Autodesk Fusion 360 part; units mm, degrees
note: some values were not read from the file. Chosen so that the rebuilt part matches the saved one: a direction. Set by a fixed rule: which sketch regions a step uses; which face or edge a step refers to.
(part 4 of 6)
  line L915 (71.0316, -22.4896) -> (71.0316, -29.1571)
  line L916 (71.6269, -30.7446) -> (71.6269, -26.6171)
  line L917 (71.6269, -25.0296) -> (71.6269, -18.3621)
  line L918 (71.6269, -16.7746) -> (71.6269, -10.1071)
  line L919 (71.6269, -8.5196) -> (71.6269, -4.3921)
  line L920 (72.2223, -5.9796) -> (72.2223, -12.6471)
  line L921 (72.2223, -14.2346) -> (72.2223, -20.9021)
  line L922 (72.2223, -22.4896) -> (72.2223, -29.1571)
  line L923 (72.8176, -30.7446) -> (72.8176, -26.6171)
  line L924 (72.8176, -25.0296) -> (72.8176, -18.3621)
  line L925 (72.8176, -16.7746) -> (72.8176, -10.1071)
  line L926 (72.8176, -8.5196) -> (72.8176, -4.3921)
  line L927 (73.4129, -5.9796) -> (73.4129, -12.6471)
  line L928 (73.4129, -14.2346) -> (73.4129, -20.9021)
  line L929 (73.4129, -22.4896) -> (73.4129, -29.1571)
  line L930 (74.0082, -30.7446) -> (74.0082, -26.6171)
  line L931 (74.0082, -25.0296) -> (74.0082, -18.3621)
  line L932 (74.0082, -16.7746) -> (74.0082, -10.1071)
  line L933 (74.0082, -8.5196) -> (74.0082, -4.3921)
  line L934 (74.6035, -5.9796) -> (74.6035, -12.6471)
  line L935 (74.6035, -14.2346) -> (74.6035, -20.9021)
  line L936 (74.6035, -22.4896) -> (74.6035, -29.1571)
  line L937 (75.1988, -30.7446) -> (75.1988, -26.6171)
  line L938 (75.1988, -25.0296) -> (75.1988, -18.3621)
  line L939 (75.1988, -16.7746) -> (75.1988, -10.1071)
  line L940 (75.1988, -8.5196) -> (75.1988, -4.3921)
  line L941 (75.7941, -5.9796) -> (75.7941, -12.6471)
  line L942 (75.7941, -14.2346) -> (75.7941, -20.9021)
  line L943 (75.7941, -22.4896) -> (75.7941, -29.1571)
  line L944 (76.3894, -30.7446) -> (76.3894, -26.6171)
  line L945 (76.3894, -25.0296) -> (76.3894, -18.3621)
  line L946 (76.3894, -16.7746) -> (76.3894, -10.1071)
  line L947 (76.3894, -8.5196) -> (76.3894, -4.3921)
  line L948 (76.9848, -5.9796) -> (76.9848, -12.6471)
  line L949 (76.9848, -14.2346) -> (76.9848, -20.9021)
  line L950 (76.9848, -22.4896) -> (76.9848, -29.1571)
  line L951 (77.5801, -30.7446) -> (77.5801, -26.6171)
  line L952 (77.5801, -25.0296) -> (77.5801, -18.3621)
  line L953 (77.5801, -16.7746) -> (77.5801, -10.1071)
  line L954 (77.5801, -8.5196) -> (77.5801, -4.3921)
  line L955 (78.1754, -5.9796) -> (78.1754, -12.6471)
  line L956 (78.1754, -14.2346) -> (78.1754, -20.9021)
  line L957 (78.1754, -22.4896) -> (78.1754, -29.1571)
  line L958 (78.7707, -30.7446) -> (78.7707, -26.6171)
  line L959 (78.7707, -25.0296) -> (78.7707, -18.3621)
  line L960 (78.7707, -16.7746) -> (78.7707, -10.1071)
  line L961 (78.7707, -8.5196) -> (78.7707, -4.3921)
  line L962 (79.366, -5.9796) -> (79.366, -12.6471)
  line L963 (79.366, -14.2346) -> (79.366, -20.9021)
  line L964 (79.366, -22.4896) -> (79.366, -29.1571)
  line L965 (79.9613, -30.7446) -> (79.9613, -26.6171)
  line L966 (79.9613, -25.0296) -> (79.9613, -18.3621)
  line L967 (79.9613, -16.7746) -> (79.9613, -10.1071)
  line L968 (79.9613, -8.5196) -> (79.9613, -4.3921)
  line L969 (80.5566, -5.9796) -> (80.5566, -12.6471)
  line L970 (80.5566, -14.2346) -> (80.5566, -20.9021)
  line L971 (80.5566, -22.4896) -> (80.5566, -29.1571)
  line L972 (81.1519, -30.7446) -> (81.1519, -26.6171)
  line L973 (81.1519, -25.0296) -> (81.1519, -18.3621)
  line L974 (81.1519, -16.7746) -> (81.1519, -10.1071)
  line L975 (81.1519, -8.5196) -> (81.1519, -4.3921)
  line L976 (81.7473, -5.9796) -> (81.7473, -12.6471)
  line L977 (81.7473, -14.2346) -> (81.7473, -20.9021)
  line L978 (81.7473, -22.4896) -> (81.7473, -29.1571)
  line L979 (82.3426, -30.7446) -> (82.3426, -26.6171)
  line L980 (82.3426, -25.0296) -> (82.3426, -18.3621)
  line L981 (82.3426, -16.7746) -> (82.3426, -10.1071)
  line L982 (82.3426, -8.5196) -> (82.3426, -4.3921)
  line L983 (82.9379, -5.9796) -> (82.9379, -12.6471)
  line L984 (82.9379, -14.2346) -> (82.9379, -20.9021)
  line L985 (82.9379, -22.4896) -> (82.9379, -29.1571)
  line L986 (83.5332, -30.7446) -> (83.5332, -26.6171)
  line L987 (83.5332, -25.0296) -> (83.5332, -18.3621)
  line L988 (83.5332, -16.7746) -> (83.5332, -10.1071)
  line L989 (83.5332, -8.5196) -> (83.5332, -4.3921)
  line L990 (84.1285, -5.9796) -> (84.1285, -12.6471)
  line L991 (84.1285, -14.2346) -> (84.1285, -20.9021)
  line L992 (84.1285, -22.4896) -> (84.1285, -29.1571)
  line L993 (84.7238, -30.7446) -> (84.7238, -26.6171)
  line L994 (84.7238, -25.0296) -> (84.7238, -18.3621)
  line L995 (84.7238, -16.7746) -> (84.7238, -10.1071)
  line L996 (84.7238, -8.5196) -> (84.7238, -4.3921)
  line L997 (85.3191, -5.9796) -> (85.3191, -12.6471)
  line L998 (85.3191, -14.2346) -> (85.3191, -20.9021)
  line L999 (85.3191, -22.4896) -> (85.3191, -29.1571)
  line L1000 (85.9144, -30.7446) -> (85.9144, -26.6171)
  line L1001 (85.9144, -25.0296) -> (85.9144, -18.3621)
  line L1002 (85.9144, -16.7746) -> (85.9144, -10.1071)
  line L1003 (85.9144, -8.5196) -> (85.9144, -4.3921)
  line L1004 (86.5098, -5.9796) -> (86.5098, -12.6471)
  line L1005 (86.5098, -14.2346) -> (86.5098, -20.9021)
  line L1006 (86.5098, -22.4896) -> (86.5098, -29.1571)
  line L1007 (87.1051, -30.7446) -> (87.1051, -26.6171)
  line L1008 (87.1051, -25.0296) -> (87.1051, -18.3621)
  line L1009 (87.1051, -16.7746) -> (87.1051, -10.1071)
  line L1010 (87.1051, -8.5196) -> (87.1051, -4.3921)
  line L1011 (87.7004, -5.9796) -> (87.7004, -12.6471)
  line L1012 (87.7004, -14.2346) -> (87.7004, -20.9021)
  line L1013 (87.7004, -22.4896) -> (87.7004, -29.1571)
  line L1014 (88.2957, -30.7446) -> (88.2957, -26.6171)
  line L1015 (88.2957, -25.0296) -> (88.2957, -18.3621)
  line L1016 (88.2957, -16.7746) -> (88.2957, -10.1071)
  line L1017 (88.2957, -8.5196) -> (88.2957, -4.3921)
  line L1018 (88.891, -5.9796) -> (88.891, -12.6471)
  line L1019 (88.891, -14.2346) -> (88.891, -20.9021)
  line L1020 (88.891, -22.4896) -> (88.891, -29.1571)
  line L1021 (89.4863, -30.7446) -> (89.4863, -26.6171)
  line L1022 (89.4863, -25.0296) -> (89.4863, -18.3621)
  line L1023 (89.4863, -16.7746) -> (89.4863, -10.1071)
  line L1024 (89.4863, -8.5196) -> (89.4863, -4.3921)
  line L1025 (90.0816, -5.9796) -> (90.0816, -12.6471)
  line L1026 (90.0816, -14.2346) -> (90.0816, -20.9021)
  line L1027 (90.0816, -22.4896) -> (90.0816, -29.1571)
  line L1028 (90.6769, -30.7446) -> (90.6769, -26.6171)
  line L1029 (90.6769, -25.0296) -> (90.6769, -18.3621)
  line L1030 (90.6769, -16.7746) -> (90.6769, -10.1071)
  line L1031 (90.6769, -8.5196) -> (90.6769, -4.3921)
  line L1032 (91.2723, -5.9796) -> (91.2723, -12.6471)
  line L1033 (91.2723, -14.2346) -> (91.2723, -20.9021)
  line L1034 (91.2723, -22.4896) -> (91.2723, -29.1571)
  line L1035 (91.8676, -30.7446) -> (91.8676, -26.6171)
  line L1036 (91.8676, -25.0296) -> (91.8676, -18.3621)
  line L1037 (91.8676, -16.7746) -> (91.8676, -10.1071)
  line L1038 (91.8676, -8.5196) -> (91.8676, -4.3921)
  line L1039 (93.7503, -30.7446) -> (95.3378, -30.7446)
  spline S766 degree 3 poles (95.3378, -30.7446) (95.3524, -30.7446) (95.3643, -30.7327) (95.3643, -30.7181) knots 0 0 0 0 1 1 1 1
  line L1040 (95.3643, -30.7181) -> (95.3643, -6.006)
  spline S767 degree 3 poles (95.3643, -6.006) (95.3643, -5.9915) (95.3524, -5.9796) (95.3378, -5.9796) knots 0 0 0 0 1 1 1 1
  line L1041 (95.3378, -5.9796) -> (93.7503, -5.9796)
  spline S768 degree 3 poles (93.7503, -5.9796) (93.7358, -5.9796) (93.7239, -5.9915) (93.7239, -6.006) knots 0 0 0 0 1 1 1 1
  line L1042 (93.7239, -6.006) -> (93.7239, -6.4294)
  spline S769 degree 3 poles (93.7239, -6.4294) (93.7239, -6.4558) (93.7503, -6.4294) (93.7239, -6.4294) knots 0 0 0 0 1 1 1 1
  line L1043 (93.7239, -6.4294) -> (92.9566, -6.4294)
  spline S770 degree 3 poles (92.9566, -6.4294) (92.942, -6.4294) (92.9301, -6.4413) (92.9301, -6.4558) knots 0 0 0 0 1 1 1 1
  line L1044 (92.9301, -6.4558) -> (92.9301, -8.0433)
  spline S771 degree 3 poles (92.9301, -8.0433) (92.9301, -8.0579) (92.942, -8.0698) (92.9566, -8.0698) knots 0 0 0 0 1 1 1 1
  line L1045 (92.9566, -8.0698) -> (93.7239, -8.0698)
  spline S772 degree 3 poles (93.7239, -8.0698) (93.7503, -8.0698) (93.7239, -8.0433) (93.7239, -8.0698) knots 0 0 0 0 1 1 1 1
  line L1046 (93.7239, -8.0698) -> (93.7239, -9.6044)
  spline S773 degree 3 poles (93.7239, -9.6044) (93.7239, -9.6308) (93.7503, -9.6044) (93.7239, -9.6044) knots 0 0 0 0 1 1 1 1
  line L1047 (93.7239, -9.6044) -> (92.9566, -9.6044)
  spline S774 degree 3 poles (92.9566, -9.6044) (92.942, -9.6044) (92.9301, -9.6163) (92.9301, -9.6308) knots 0 0 0 0 1 1 1 1
  line L1048 (92.9301, -9.6308) -> (92.9301, -11.2183)
  spline S775 degree 3 poles (92.9301, -11.2183) (92.9301, -11.2329) (92.942, -11.2448) (92.9566, -11.2448) knots 0 0 0 0 1 1 1 1
  line L1049 (92.9566, -11.2448) -> (93.7239, -11.2448)
  spline S776 degree 3 poles (93.7239, -11.2448) (93.7503, -11.2448) (93.7239, -11.2183) (93.7239, -11.2448) knots 0 0 0 0 1 1 1 1
  line L1050 (93.7239, -11.2448) -> (93.7239, -12.7794)
  spline S777 degree 3 poles (93.7239, -12.7794) (93.7239, -12.8058) (93.7503, -12.7794) (93.7239, -12.7794) knots 0 0 0 0 1 1 1 1
  line L1051 (93.7239, -12.7794) -> (92.9566, -12.7794)
  spline S778 degree 3 poles (92.9566, -12.7794) (92.942, -12.7794) (92.9301, -12.7913) (92.9301, -12.8058) knots 0 0 0 0 1 1 1 1
  line L1052 (92.9301, -12.8058) -> (92.9301, -14.3933)
  spline S779 degree 3 poles (92.9301, -14.3933) (92.9301, -14.4079) (92.942, -14.4198) (92.9566, -14.4198) knots 0 0 0 0 1 1 1 1
  line L1053 (92.9566, -14.4198) -> (93.7239, -14.4198)
  spline S780 degree 3 poles (93.7239, -14.4198) (93.7503, -14.4198) (93.7239, -14.3933) (93.7239, -14.4198) knots 0 0 0 0 1 1 1 1
  line L1054 (93.7239, -14.4198) -> (93.7239, -15.9544)
  spline S781 degree 3 poles (93.7239, -15.9544) (93.7239, -15.9808) (93.7503, -15.9544) (93.7239, -15.9544) knots 0 0 0 0 1 1 1 1
  line L1055 (93.7239, -15.9544) -> (92.9566, -15.9544)
  spline S782 degree 3 poles (92.9566, -15.9544) (92.942, -15.9544) (92.9301, -15.9663) (92.9301, -15.9808) knots 0 0 0 0 1 1 1 1
  line L1056 (92.9301, -15.9808) -> (92.9301, -17.5683)
  spline S783 degree 3 poles (92.9301, -17.5683) (92.9301, -17.5829) (92.942, -17.5948) (92.9566, -17.5948) knots 0 0 0 0 1 1 1 1
  line L1057 (92.9566, -17.5948) -> (93.7239, -17.5948)
  spline S784 degree 3 poles (93.7239, -17.5948) (93.7503, -17.5948) (93.7239, -17.5683) (93.7239, -17.5948) knots 0 0 0 0 1 1 1 1
  line L1058 (93.7239, -17.5948) -> (93.7239, -19.1294)
  spline S785 degree 3 poles (93.7239, -19.1294) (93.7239, -19.1558) (93.7503, -19.1294) (93.7239, -19.1294) knots 0 0 0 0 1 1 1 1
  line L1059 (93.7239, -19.1294) -> (92.9566, -19.1294)
  spline S786 degree 3 poles (92.9566, -19.1294) (92.942, -19.1294) (92.9301, -19.1413) (92.9301, -19.1558) knots 0 0 0 0 1 1 1 1
  line L1060 (92.9301, -19.1558) -> (92.9301, -20.7433)
  spline S787 degree 3 poles (92.9301, -20.7433) (92.9301, -20.7579) (92.942, -20.7698) (92.9566, -20.7698) knots 0 0 0 0 1 1 1 1
  line L1061 (92.9566, -20.7698) -> (93.7239, -20.7698)
  spline S788 degree 3 poles (93.7239, -20.7698) (93.7503, -20.7698) (93.7239, -20.7433) (93.7239, -20.7698) knots 0 0 0 0 1 1 1 1
  line L1062 (93.7239, -20.7698) -> (93.7239, -22.3044)
  spline S789 degree 3 poles (93.7239, -22.3044) (93.7239, -22.3308) (93.7503, -22.3044) (93.7239, -22.3044) knots 0 0 0 0 1 1 1 1
  line L1063 (93.7239, -22.3044) -> (92.9566, -22.3044)
  spline S790 degree 3 poles (92.9566, -22.3044) (92.942, -22.3044) (92.9301, -22.3163) (92.9301, -22.3308) knots 0 0 0 0 1 1 1 1
  line L1064 (92.9301, -22.3308) -> (92.9301, -23.9183)
  spline S791 degree 3 poles (92.9301, -23.9183) (92.9301, -23.9329) (92.942, -23.9448) (92.9566, -23.9448) knots 0 0 0 0 1 1 1 1
  line L1065 (92.9566, -23.9448) -> (93.7239, -23.9448)
  spline S792 degree 3 poles (93.7239, -23.9448) (93.7503, -23.9448) (93.7239, -23.9183) (93.7239, -23.9448) knots 0 0 0 0 1 1 1 1
  line L1066 (93.7239, -23.9448) -> (93.7239, -25.4794)
  spline S793 degree 3 poles (93.7239, -25.4794) (93.7239, -25.5058) (93.7503, -25.4794) (93.7239, -25.4794) knots 0 0 0 0 1 1 1 1
  line L1067 (93.7239, -25.4794) -> (92.9566, -25.4794)
  spline S794 degree 3 poles (92.9566, -25.4794) (92.942, -25.4794) (92.9301, -25.4913) (92.9301, -25.5058) knots 0 0 0 0 1 1 1 1
  line L1068 (92.9301, -25.5058) -> (92.9301, -27.0933)
  spline S795 degree 3 poles (92.9301, -27.0933) (92.9301, -27.1079) (92.942, -27.1198) (92.9566, -27.1198) knots 0 0 0 0 1 1 1 1
  line L1069 (92.9566, -27.1198) -> (93.7239, -27.1198)
  spline S796 degree 3 poles (93.7239, -27.1198) (93.7503, -27.1198) (93.7239, -27.0933) (93.7239, -27.1198) knots 0 0 0 0 1 1 1 1
  line L1070 (93.7239, -27.1198) -> (93.7239, -28.6544)
  spline S797 degree 3 poles (93.7239, -28.6544) (93.7239, -28.6808) (93.7503, -28.6544) (93.7239, -28.6544) knots 0 0 0 0 1 1 1 1
  line L1071 (93.7239, -28.6544) -> (92.9566, -28.6544)
  spline S798 degree 3 poles (92.9566, -28.6544) (92.942, -28.6544) (92.9301, -28.6663) (92.9301, -28.6808) knots 0 0 0 0 1 1 1 1
  line L1072 (92.9301, -28.6808) -> (92.9301, -30.2683)
  spline S799 degree 3 poles (92.9301, -30.2683) (92.9301, -30.2829) (92.942, -30.2948) (92.9566, -30.2948) knots 0 0 0 0 1 1 1 1
  line L1073 (92.9566, -30.2948) -> (93.7239, -30.2948)
  spline S800 degree 3 poles (93.7239, -30.2948) (93.7503, -30.2948) (93.7239, -30.2683) (93.7239, -30.2948) knots 0 0 0 0 1 1 1 1
  line L1074 (93.7239, -30.2948) -> (93.7239, -30.7181)
  spline S801 degree 3 poles (93.7239, -30.7181) (93.7239, -30.7327) (93.7358, -30.7446) (93.7503, -30.7446) knots 0 0 0 0 1 1 1 1
  line L1075 (95.7876, -29.9508) -> (96.8195, -29.9508)
  spline S802 degree 3 poles (96.8195, -29.9508) (96.846, -29.9508) (96.8195, -29.9244) (96.8195, -29.9508) knots 0 0 0 0 1 1 1 1
  line L1076 (96.8195, -29.9508) -> (96.8195, -30.7181)
  spline S803 degree 3 poles (96.8195, -30.7181) (96.8195, -30.7327) (96.8314, -30.7446) (96.846, -30.7446) knots 0 0 0 0 1 1 1 1
  line L1077 (96.846, -30.7446) -> (98.4335, -30.7446)
  spline S804 degree 3 poles (98.4335, -30.7446) (98.448, -30.7446) (98.4599, -30.7327) (98.4599, -30.7181) knots 0 0 0 0 1 1 1 1
  line L1078 (98.4599, -30.7181) -> (98.4599, -29.9508)
  spline S805 degree 3 poles (98.4599, -29.9508) (98.4599, -29.9244) (98.4335, -29.9508) (98.4599, -29.9508) knots 0 0 0 0 1 1 1 1
  line L1079 (98.4599, -29.9508) -> (99.9945, -29.9508)
  spline S806 degree 3 poles (99.9945, -29.9508) (100.021, -29.9508) (99.9945, -29.9244) (99.9945, -29.9508) knots 0 0 0 0 1 1 1 1
  line L1080 (99.9945, -29.9508) -> (99.9945, -30.7181)
  spline S807 degree 3 poles (99.9945, -30.7181) (99.9945, -30.7327) (100.0064, -30.7446) (100.021, -30.7446) knots 0 0 0 0 1 1 1 1
  line L1081 (100.021, -30.7446) -> (101.6085, -30.7446)
  spline S808 degree 3 poles (101.6085, -30.7446) (101.623, -30.7446) (101.6349, -30.7327) (101.6349, -30.7181) knots 0 0 0 0 1 1 1 1
  line L1082 (101.6349, -30.7181) -> (101.6349, -29.9508)
  spline S809 degree 3 poles (101.6349, -29.9508) (101.6349, -29.9244) (101.6085, -29.9508) (101.6349, -29.9508) knots 0 0 0 0 1 1 1 1
  line L1083 (101.6349, -29.9508) -> (103.1695, -29.9508)
  spline S810 degree 3 poles (103.1695, -29.9508) (103.196, -29.9508) (103.1695, -29.9244) (103.1695, -29.9508) knots 0 0 0 0 1 1 1 1
  line L1084 (103.1695, -29.9508) -> (103.1695, -30.7181)
  spline S811 degree 3 poles (103.1695, -30.7181) (103.1695, -30.7327) (103.1814, -30.7446) (103.196, -30.7446) knots 0 0 0 0 1 1 1 1
  line L1085 (103.196, -30.7446) -> (104.7835, -30.7446)
  spline S812 degree 3 poles (104.7835, -30.7446) (104.798, -30.7446) (104.8099, -30.7327) (104.8099, -30.7181) knots 0 0 0 0 1 1 1 1
  line L1086 (104.8099, -30.7181) -> (104.8099, -29.9508)
  spline S813 degree 3 poles (104.8099, -29.9508) (104.8099, -29.9244) (104.7835, -29.9508) (104.8099, -29.9508) knots 0 0 0 0 1 1 1 1
  line L1087 (104.8099, -29.9508) -> (106.3445, -29.9508)
  spline S814 degree 3 poles (106.3445, -29.9508) (106.371, -29.9508) (106.3445, -29.9244) (106.3445, -29.9508) knots 0 0 0 0 1 1 1 1
  line L1088 (106.3445, -29.9508) -> (106.3445, -30.7181)
  spline S815 degree 3 poles (106.3445, -30.7181) (106.3445, -30.7327) (106.3564, -30.7446) (106.371, -30.7446) knots 0 0 0 0 1 1 1 1
  line L1089 (106.371, -30.7446) -> (107.9585, -30.7446)
  spline S816 degree 3 poles (107.9585, -30.7446) (107.973, -30.7446) (107.9849, -30.7327) (107.9849, -30.7181) knots 0 0 0 0 1 1 1 1
  line L1090 (107.9849, -30.7181) -> (107.9849, -29.9508)
  spline S817 degree 3 poles (107.9849, -29.9508) (107.9849, -29.9244) (107.9585, -29.9508) (107.9849, -29.9508) knots 0 0 0 0 1 1 1 1
  line L1091 (107.9849, -29.9508) -> (109.5195, -29.9508)
  spline S818 degree 3 poles (109.5195, -29.9508) (109.546, -29.9508) (109.5195, -29.9244) (109.5195, -29.9508) knots 0 0 0 0 1 1 1 1
  line L1092 (109.5195, -29.9508) -> (109.5195, -30.7181)
  spline S819 degree 3 poles (109.5195, -30.7181) (109.5195, -30.7327) (109.5314, -30.7446) (109.546, -30.7446) knots 0 0 0 0 1 1 1 1
  line L1093 (109.546, -30.7446) -> (111.1335, -30.7446)
  spline S820 degree 3 poles (111.1335, -30.7446) (111.148, -30.7446) (111.1599, -30.7327) (111.1599, -30.7181) knots 0 0 0 0 1 1 1 1
  line L1094 (111.1599, -30.7181) -> (111.1599, -29.9508)
  spline S821 degree 3 poles (111.1599, -29.9508) (111.1599, -29.9244) (111.1335, -29.9508) (111.1599, -29.9508) knots 0 0 0 0 1 1 1 1
  line L1095 (111.1599, -29.9508) -> (112.6945, -29.9508)
  spline S822 degree 3 poles (112.6945, -29.9508) (112.721, -29.9508) (112.6945, -29.9244) (112.6945, -29.9508) knots 0 0 0 0 1 1 1 1
  line L1096 (112.6945, -29.9508) -> (112.6945, -30.7181)
  spline S823 degree 3 poles (112.6945, -30.7181) (112.6945, -30.7327) (112.7064, -30.7446) (112.721, -30.7446) knots 0 0 0 0 1 1 1 1
  line L1097 (112.721, -30.7446) -> (114.3085, -30.7446)
  spline S824 degree 3 poles (114.3085, -30.7446) (114.323, -30.7446) (114.3349, -30.7327) (114.3349, -30.7181) knots 0 0 0 0 1 1 1 1
  line L1098 (114.3349, -30.7181) -> (114.3349, -29.9508)
  spline S825 degree 3 poles (114.3349, -29.9508) (114.3349, -29.9244) (114.3085, -29.9508) (114.3349, -29.9508) knots 0 0 0 0 1 1 1 1
  line L1099 (114.3349, -29.9508) -> (115.8695, -29.9508)
  spline S826 degree 3 poles (115.8695, -29.9508) (115.896, -29.9508) (115.8695, -29.9244) (115.8695, -29.9508) knots 0 0 0 0 1 1 1 1
  line L1100 (115.8695, -29.9508) -> (115.8695, -30.7181)
  spline S827 degree 3 poles (115.8695, -30.7181) (115.8695, -30.7327) (115.8814, -30.7446) (115.896, -30.7446) knots 0 0 0 0 1 1 1 1
  line L1101 (115.896, -30.7446) -> (117.4835, -30.7446)
  spline S828 degree 3 poles (117.4835, -30.7446) (117.498, -30.7446) (117.5099, -30.7327) (117.5099, -30.7181) knots 0 0 0 0 1 1 1 1
  line L1102 (117.5099, -30.7181) -> (117.5099, -29.9508)
  spline S829 degree 3 poles (117.5099, -29.9508) (117.5099, -29.9244) (117.4835, -29.9508) (117.5099, -29.9508) knots 0 0 0 0 1 1 1 1
  line L1103 (117.5099, -29.9508) -> (119.0445, -29.9508)
  spline S830 degree 3 poles (119.0445, -29.9508) (119.071, -29.9508) (119.0445, -29.9244) (119.0445, -29.9508) knots 0 0 0 0 1 1 1 1
  line L1104 (119.0445, -29.9508) -> (119.0445, -30.7181)
  spline S831 degree 3 poles (119.0445, -30.7181) (119.0445, -30.7327) (119.0564, -30.7446) (119.071, -30.7446) knots 0 0 0 0 1 1 1 1
  line L1105 (119.071, -30.7446) -> (120.6585, -30.7446)
  spline S832 degree 3 poles (120.6585, -30.7446) (120.673, -30.7446) (120.6849, -30.7327) (120.6849, -30.7181) knots 0 0 0 0 1 1 1 1
  line L1106 (120.6849, -30.7181) -> (120.6849, -29.9508)
  spline S833 degree 3 poles (120.6849, -29.9508) (120.6849, -29.9244) (120.6585, -29.9508) (120.6849, -29.9508) knots 0 0 0 0 1 1 1 1
  line L1107 (120.6849, -29.9508) -> (122.2195, -29.9508)
  spline S834 degree 3 poles (122.2195, -29.9508) (122.246, -29.9508) (122.2195, -29.9244) (122.2195, -29.9508) knots 0 0 0 0 1 1 1 1
  line L1108 (122.2195, -29.9508) -> (122.2195, -30.7181)
  spline S835 degree 3 poles (122.2195, -30.7181) (122.2195, -30.7327) (122.2314, -30.7446) (122.246, -30.7446) knots 0 0 0 0 1 1 1 1
  line L1109 (122.246, -30.7446) -> (123.8335, -30.7446)
  spline S836 degree 3 poles (123.8335, -30.7446) (123.848, -30.7446) (123.8599, -30.7327) (123.8599, -30.7181) knots 0 0 0 0 1 1 1 1
  line L1110 (123.8599, -30.7181) -> (123.8599, -29.9508)
  spline S837 degree 3 poles (123.8599, -29.9508) (123.8599, -29.9244) (123.8335, -29.9508) (123.8599, -29.9508) knots 0 0 0 0 1 1 1 1
  line L1111 (123.8599, -29.9508) -> (124.8918, -29.9508)
  line L1112 (124.8918, -29.9508) -> (124.7907, -29.9508)
  spline S838 degree 3 poles (124.7907, -29.9508) (124.8055, -29.9508) (124.8172, -29.9389) (124.8172, -29.9244) knots 0 0 0 0 1 1 1 1
  line L1113 (124.8172, -29.9244) -> (124.8172, -27.0404)
  spline S839 degree 3 poles (124.8172, -27.0404) (124.8172, -27.014) (124.7907, -27.0404) (124.8172, -27.0404) knots 0 0 0 0 1 1 1 1
  line L1114 (124.8172, -27.0404) -> (124.9963, -27.0404)
  spline S840 degree 3 poles (124.9963, -27.0404) (125.0109, -27.0404) (125.0228, -27.0285) (125.0228, -27.014) knots 0 0 0 0 1 1 1 1
  line L1115 (125.0228, -27.014) -> (125.0228, -25.4265)
  spline S841 degree 3 poles (125.0228, -25.4265) (125.0228, -25.4119) (125.0109, -25.4) (124.9963, -25.4) knots 0 0 0 0 1 1 1 1
  line L1116 (124.9963, -25.4) -> (124.8172, -25.4)
  spline S842 degree 3 poles (124.8172, -25.4) (124.7907, -25.4) (124.8172, -25.4265) (124.8172, -25.4) knots 0 0 0 0 1 1 1 1
  line L1117 (124.8172, -25.4) -> (124.8172, -23.8654)
  spline S843 degree 3 poles (124.8172, -23.8654) (124.8172, -23.839) (124.7907, -23.8654) (124.8172, -23.8654) knots 0 0 0 0 1 1 1 1
  line L1118 (124.8172, -23.8654) -> (124.9963, -23.8654)
  spline S844 degree 3 poles (124.9963, -23.8654) (125.0109, -23.8654) (125.0228, -23.8535) (125.0228, -23.839) knots 0 0 0 0 1 1 1 1
  line L1119 (125.0228, -23.839) -> (125.0228, -22.2515)
  spline S845 degree 3 poles (125.0228, -22.2515) (125.0228, -22.2369) (125.0109, -22.225) (124.9963, -22.225) knots 0 0 0 0 1 1 1 1
  line L1120 (124.9963, -22.225) -> (124.8172, -22.225)
  spline S846 degree 3 poles (124.8172, -22.225) (124.7907, -22.225) (124.8172, -22.2515) (124.8172, -22.225) knots 0 0 0 0 1 1 1 1
  line L1121 (124.8172, -22.225) -> (124.8172, -20.6904)
  spline S847 degree 3 poles (124.8172, -20.6904) (124.8172, -20.664) (124.7907, -20.6904) (124.8172, -20.6904) knots 0 0 0 0 1 1 1 1
  line L1122 (124.8172, -20.6904) -> (124.9963, -20.6904)
  spline S848 degree 3 poles (124.9963, -20.6904) (125.0109, -20.6904) (125.0228, -20.6785) (125.0228, -20.664) knots 0 0 0 0 1 1 1 1
  line L1123 (125.0228, -20.664) -> (125.0228, -19.0765)
  spline S849 degree 3 poles (125.0228, -19.0765) (125.0228, -19.0619) (125.0109, -19.05) (124.9963, -19.05) knots 0 0 0 0 1 1 1 1
  line L1124 (124.9963, -19.05) -> (124.8172, -19.05)
  spline S850 degree 3 poles (124.8172, -19.05) (124.7907, -19.05) (124.8172, -19.0765) (124.8172, -19.05) knots 0 0 0 0 1 1 1 1
  line L1125 (124.8172, -19.05) -> (124.8172, -17.5154)
  spline S851 degree 3 poles (124.8172, -17.5154) (124.8172, -17.489) (124.7907, -17.5154) (124.8172, -17.5154) knots 0 0 0 0 1 1 1 1
  line L1126 (124.8172, -17.5154) -> (124.9963, -17.5154)
  spline S852 degree 3 poles (124.9963, -17.5154) (125.0109, -17.5154) (125.0228, -17.5035) (125.0228, -17.489) knots 0 0 0 0 1 1 1 1
  line L1127 (125.0228, -17.489) -> (125.0228, -15.9015)
  spline S853 degree 3 poles (125.0228, -15.9015) (125.0228, -15.8869) (125.0109, -15.875) (124.9963, -15.875) knots 0 0 0 0 1 1 1 1
  line L1128 (124.9963, -15.875) -> (124.8172, -15.875)
  spline S854 degree 3 poles (124.8172, -15.875) (124.7907, -15.875) (124.8172, -15.9015) (124.8172, -15.875) knots 0 0 0 0 1 1 1 1
  line L1129 (124.8172, -15.875) -> (124.8172, -14.3404)
  spline S855 degree 3 poles (124.8172, -14.3404) (124.8172, -14.314) (124.7907, -14.3404) (124.8172, -14.3404) knots 0 0 0 0 1 1 1 1
  line L1130 (124.8172, -14.3404) -> (124.9963, -14.3404)
  spline S856 degree 3 poles (124.9963, -14.3404) (125.0109, -14.3404) (125.0228, -14.3285) (125.0228, -14.314) knots 0 0 0 0 1 1 1 1
  line L1131 (125.0228, -14.314) -> (125.0228, -12.7265)
  spline S857 degree 3 poles (125.0228, -12.7265) (125.0228, -12.7119) (125.0109, -12.7) (124.9963, -12.7) knots 0 0 0 0 1 1 1 1
  line L1132 (124.9963, -12.7) -> (124.8172, -12.7)
  spline S858 degree 3 poles (124.8172, -12.7) (124.7907, -12.7) (124.8172, -12.7265) (124.8172, -12.7) knots 0 0 0 0 1 1 1 1
  line L1133 (124.8172, -12.7) -> (124.8172, -11.1654)
  spline S859 degree 3 poles (124.8172, -11.1654) (124.8172, -11.139) (124.7907, -11.1654) (124.8172, -11.1654) knots 0 0 0 0 1 1 1 1
  line L1134 (124.8172, -11.1654) -> (124.9963, -11.1654)
  spline S860 degree 3 poles (124.9963, -11.1654) (125.0109, -11.1654) (125.0228, -11.1535) (125.0228, -11.139) knots 0 0 0 0 1 1 1 1
  line L1135 (125.0228, -11.139) -> (125.0228, -9.5515)
  spline S861 degree 3 poles (125.0228, -9.5515) (125.0228, -9.5369) (125.0109, -9.525) (124.9963, -9.525) knots 0 0 0 0 1 1 1 1
  line L1136 (124.9963, -9.525) -> (124.8172, -9.525)
  spline S862 degree 3 poles (124.8172, -9.525) (124.7907, -9.525) (124.8172, -9.5515) (124.8172, -9.525) knots 0 0 0 0 1 1 1 1
  line L1137 (124.8172, -9.525) -> (124.8172, -7.9904)
  spline S863 degree 3 poles (124.8172, -7.9904) (124.8172, -7.964) (124.7907, -7.9904) (124.8172, -7.9904) knots 0 0 0 0 1 1 1 1
  line L1138 (124.8172, -7.9904) -> (124.9963, -7.9904)
  spline S864 degree 3 poles (124.9963, -7.9904) (125.0109, -7.9904) (125.0228, -7.9785) (125.0228, -7.964) knots 0 0 0 0 1 1 1 1
  line L1139 (125.0228, -7.964) -> (125.0228, -6.3765)
  spline S865 degree 3 poles (125.0228, -6.3765) (125.0228, -6.3619) (125.0109, -6.35) (124.9963, -6.35) knots 0 0 0 0 1 1 1 1
  line L1140 (124.9963, -6.35) -> (124.8172, -6.35)
  spline S866 degree 3 poles (124.8172, -6.35) (124.7907, -6.35) (124.8172, -6.3765) (124.8172, -6.35) knots 0 0 0 0 1 1 1 1
  line L1141 (124.8172, -6.35) -> (124.8172, -3.466)
  spline S867 degree 3 poles (124.8172, -3.466) (124.8172, -3.4515) (124.8055, -3.4396) (124.7907, -3.4396) knots 0 0 0 0 1 1 1 1
  line L1142 (124.7907, -3.4396) -> (124.8918, -3.4396)
  line L1143 (124.8918, -3.4396) -> (123.8599, -3.4396)
  spline S868 degree 3 poles (123.8599, -3.4396) (123.8335, -3.4396) (123.8599, -3.466) (123.8599, -3.4396) knots 0 0 0 0 1 1 1 1
  line L1144 (123.8599, -3.4396) -> (123.8599, -2.6723)
  spline S869 degree 3 poles (123.8599, -2.6723) (123.8599, -2.6577) (123.848, -2.6458) (123.8335, -2.6458) knots 0 0 0 0 1 1 1 1
  line L1145 (123.8335, -2.6458) -> (122.246, -2.6458)
  spline S870 degree 3 poles (122.246, -2.6458) (122.2314, -2.6458) (122.2195, -2.6577) (122.2195, -2.6723) knots 0 0 0 0 1 1 1 1
  line L1146 (122.2195, -2.6723) -> (122.2195, -3.4396)
  spline S871 degree 3 poles (122.2195, -3.4396) (122.2195, -3.466) (122.246, -3.4396) (122.2195, -3.4396) knots 0 0 0 0 1 1 1 1
  line L1147 (122.2195, -3.4396) -> (120.6849, -3.4396)
  spline S872 degree 3 poles (120.6849, -3.4396) (120.6585, -3.4396) (120.6849, -3.466) (120.6849, -3.4396) knots 0 0 0 0 1 1 1 1
  line L1148 (120.6849, -3.4396) -> (120.6849, -2.6723)
  spline S873 degree 3 poles (120.6849, -2.6723) (120.6849, -2.6577) (120.673, -2.6458) (120.6585, -2.6458) knots 0 0 0 0 1 1 1 1
  line L1149 (120.6585, -2.6458) -> (119.071, -2.6458)
  spline S874 degree 3 poles (119.071, -2.6458) (119.0564, -2.6458) (119.0445, -2.6577) (119.0445, -2.6723) knots 0 0 0 0 1 1 1 1
  line L1150 (119.0445, -2.6723) -> (119.0445, -3.4396)
  spline S875 degree 3 poles (119.0445, -3.4396) (119.0445, -3.466) (119.071, -3.4396) (119.0445, -3.4396) knots 0 0 0 0 1 1 1 1
  line L1151 (119.0445, -3.4396) -> (117.5099, -3.4396)
  spline S876 degree 3 poles (117.5099, -3.4396) (117.4835, -3.4396) (117.5099, -3.466) (117.5099, -3.4396) knots 0 0 0 0 1 1 1 1
  line L1152 (117.5099, -3.4396) -> (117.5099, -2.6723)
  spline S877 degree 3 poles (117.5099, -2.6723) (117.5099, -2.6577) (117.498, -2.6458) (117.4835, -2.6458) knots 0 0 0 0 1 1 1 1
  line L1153 (117.4835, -2.6458) -> (115.896, -2.6458)
  spline S878 degree 3 poles (115.896, -2.6458) (115.8814, -2.6458) (115.8695, -2.6577) (115.8695, -2.6723) knots 0 0 0 0 1 1 1 1
  line L1154 (115.8695, -2.6723) -> (115.8695, -3.4396)
  spline S879 degree 3 poles (115.8695, -3.4396) (115.8695, -3.466) (115.896, -3.4396) (115.8695, -3.4396) knots 0 0 0 0 1 1 1 1
  line L1155 (115.8695, -3.4396) -> (114.3349, -3.4396)
  spline S880 degree 3 poles (114.3349, -3.4396) (114.3085, -3.4396) (114.3349, -3.466) (114.3349, -3.4396) knots 0 0 0 0 1 1 1 1
  line L1156 (114.3349, -3.4396) -> (114.3349, -2.6723)
  spline S881 degree 3 poles (114.3349, -2.6723) (114.3349, -2.6577) (114.323, -2.6458) (114.3085, -2.6458) knots 0 0 0 0 1 1 1 1
  line L1157 (114.3085, -2.6458) -> (112.721, -2.6458)
  spline S882 degree 3 poles (112.721, -2.6458) (112.7064, -2.6458) (112.6945, -2.6577) (112.6945, -2.6723) knots 0 0 0 0 1 1 1 1
  line L1158 (112.6945, -2.6723) -> (112.6945, -3.4396)
  spline S883 degree 3 poles (112.6945, -3.4396) (112.6945, -3.466) (112.721, -3.4396) (112.6945, -3.4396) knots 0 0 0 0 1 1 1 1
  line L1159 (112.6945, -3.4396) -> (111.1599, -3.4396)
  spline S884 degree 3 poles (111.1599, -3.4396) (111.1335, -3.4396) (111.1599, -3.466) (111.1599, -3.4396) knots 0 0 0 0 1 1 1 1
  line L1160 (111.1599, -3.4396) -> (111.1599, -2.6723)
  spline S885 degree 3 poles (111.1599, -2.6723) (111.1599, -2.6577) (111.148, -2.6458) (111.1335, -2.6458) knots 0 0 0 0 1 1 1 1
  line L1161 (111.1335, -2.6458) -> (109.546, -2.6458)
  spline S886 degree 3 poles (109.546, -2.6458) (109.5314, -2.6458) (109.5195, -2.6577) (109.5195, -2.6723) knots 0 0 0 0 1 1 1 1
  line L1162 (109.5195, -2.6723) -> (109.5195, -3.4396)
  spline S887 degree 3 poles (109.5195, -3.4396) (109.5195, -3.466) (109.546, -3.4396) (109.5195, -3.4396) knots 0 0 0 0 1 1 1 1
  line L1163 (109.5195, -3.4396) -> (107.9849, -3.4396)
  spline S888 degree 3 poles (107.9849, -3.4396) (107.9585, -3.4396) (107.9849, -3.466) (107.9849, -3.4396) knots 0 0 0 0 1 1 1 1
  line L1164 (107.9849, -3.4396) -> (107.9849, -2.6723)
  spline S889 degree 3 poles (107.9849, -2.6723) (107.9849, -2.6577) (107.973, -2.6458) (107.9585, -2.6458) knots 0 0 0 0 1 1 1 1
  line L1165 (107.9585, -2.6458) -> (106.371, -2.6458)
  spline S890 degree 3 poles (106.371, -2.6458) (106.3564, -2.6458) (106.3445, -2.6577) (106.3445, -2.6723) knots 0 0 0 0 1 1 1 1
  line L1166 (106.3445, -2.6723) -> (106.3445, -3.4396)
  spline S891 degree 3 poles (106.3445, -3.4396) (106.3445, -3.466) (106.371, -3.4396) (106.3445, -3.4396) knots 0 0 0 0 1 1 1 1
  line L1167 (106.3445, -3.4396) -> (104.8099, -3.4396)
  spline S892 degree 3 poles (104.8099, -3.4396) (104.7835, -3.4396) (104.8099, -3.466) (104.8099, -3.4396) knots 0 0 0 0 1 1 1 1
  line L1168 (104.8099, -3.4396) -> (104.8099, -2.6723)
  spline S893 degree 3 poles (104.8099, -2.6723) (104.8099, -2.6577) (104.798, -2.6458) (104.7835, -2.6458) knots 0 0 0 0 1 1 1 1
  line L1169 (104.7835, -2.6458) -> (103.196, -2.6458)
  spline S894 degree 3 poles (103.196, -2.6458) (103.1814, -2.6458) (103.1695, -2.6577) (103.1695, -2.6723) knots 0 0 0 0 1 1 1 1
  line L1170 (103.1695, -2.6723) -> (103.1695, -3.4396)
  spline S895 degree 3 poles (103.1695, -3.4396) (103.1695, -3.466) (103.196, -3.4396) (103.1695, -3.4396) knots 0 0 0 0 1 1 1 1
  line L1171 (103.1695, -3.4396) -> (101.6349, -3.4396)
  spline S896 degree 3 poles (101.6349, -3.4396) (101.6085, -3.4396) (101.6349, -3.466) (101.6349, -3.4396) knots 0 0 0 0 1 1 1 1
  line L1172 (101.6349, -3.4396) -> (101.6349, -2.6723)
  spline S897 degree 3 poles (101.6349, -2.6723) (101.6349, -2.6577) (101.623, -2.6458) (101.6085, -2.6458) knots 0 0 0 0 1 1 1 1
  line L1173 (101.6085, -2.6458) -> (100.021, -2.6458)
  spline S898 degree 3 poles (100.021, -2.6458) (100.0064, -2.6458) (99.9945, -2.6577) (99.9945, -2.6723) knots 0 0 0 0 1 1 1 1
  line L1174 (99.9945, -2.6723) -> (99.9945, -3.4396)
  spline S899 degree 3 poles (99.9945, -3.4396) (99.9945, -3.466) (100.021, -3.4396) (99.9945, -3.4396) knots 0 0 0 0 1 1 1 1
  line L1175 (99.9945, -3.4396) -> (98.4599, -3.4396)
  spline S900 degree 3 poles (98.4599, -3.4396) (98.4335, -3.4396) (98.4599, -3.466) (98.4599, -3.4396) knots 0 0 0 0 1 1 1 1
  line L1176 (98.4599, -3.4396) -> (98.4599, -2.6723)
  spline S901 degree 3 poles (98.4599, -2.6723) (98.4599, -2.6577) (98.448, -2.6458) (98.4335, -2.6458) knots 0 0 0 0 1 1 1 1
  line L1177 (98.4335, -2.6458) -> (96.846, -2.6458)
  spline S902 degree 3 poles (96.846, -2.6458) (96.8314, -2.6458) (96.8195, -2.6577) (96.8195, -2.6723) knots 0 0 0 0 1 1 1 1
  line L1178 (96.8195, -2.6723) -> (96.8195, -3.4396)
  spline S903 degree 3 poles (96.8195, -3.4396) (96.8195, -3.466) (96.846, -3.4396) (96.8195, -3.4396) knots 0 0 0 0 1 1 1 1
  line L1179 (96.8195, -3.4396) -> (95.7876, -3.4396)
  spline S904 degree 3 poles (95.7876, -3.4396) (95.7731, -3.4396) (95.7612, -3.4515) (95.7612, -3.466) knots 0 0 0 0 1 1 1 1
  line L1180 (95.7612, -3.466) -> (95.7612, -29.9244)
  spline S905 degree 3 poles (95.7612, -29.9244) (95.7612, -29.9389) (95.7731, -29.9508) (95.7876, -29.9508) knots 0 0 0 0 1 1 1 1
  line L1181 (125.5506, -29.9508) -> (126.9558, -29.9508)
  spline S906 degree 3 poles (126.9558, -29.9508) (126.9823, -29.9508) (126.9558, -29.9244) (126.9558, -29.9508) knots 0 0 0 0 1 1 1 1
  line L1182 (126.9558, -29.9508) -> (126.9558, -30.7181)
  spline S907 degree 3 poles (126.9558, -30.7181) (126.9558, -30.7327) (126.9677, -30.7446) (126.9823, -30.7446) knots 0 0 0 0 1 1 1 1
  line L1183 (126.9823, -30.7446) -> (128.5698, -30.7446)
  spline S908 degree 3 poles (128.5698, -30.7446) (128.5846, -30.7446) (128.5962, -30.7327) (128.5962, -30.7181) knots 0 0 0 0 1 1 1 1
  line L1184 (128.5962, -30.7181) -> (128.5962, -29.9508)
  spline S909 degree 3 poles (128.5962, -29.9508) (128.5962, -29.9244) (128.5698, -29.9508) (128.5962, -29.9508) knots 0 0 0 0 1 1 1 1
  line L1185 (128.5962, -29.9508) -> (130.0017, -29.9508)
  line L1186 (130.0017, -29.9508) -> (129.8175, -29.9508)
  spline S910 degree 3 poles (129.8175, -29.9508) (129.8321, -29.9508) (129.844, -29.9389) (129.844, -29.9244) knots 0 0 0 0 1 1 1 1
  line L1187 (129.844, -29.9244) -> (129.844, -27.0404)
  spline S911 degree 3 poles (129.844, -27.0404) (129.844, -27.014) (129.8175, -27.0404) (129.844, -27.0404) knots 0 0 0 0 1 1 1 1
  line L1188 (129.844, -27.0404) -> (130.2144, -27.0404)
  spline S912 degree 3 poles (130.2144, -27.0404) (130.229, -27.0404) (130.2409, -27.0285) (130.2409, -27.014) knots 0 0 0 0 1 1 1 1
  line L1189 (130.2409, -27.014) -> (130.2409, -25.4265)
  spline S913 degree 3 poles (130.2409, -25.4265) (130.2409, -25.4119) (130.229, -25.4) (130.2144, -25.4) knots 0 0 0 0 1 1 1 1
  line L1190 (130.2144, -25.4) -> (129.844, -25.4)
  spline S914 degree 3 poles (129.844, -25.4) (129.8175, -25.4) (129.844, -25.4265) (129.844, -25.4) knots 0 0 0 0 1 1 1 1
  line L1191 (129.844, -25.4) -> (129.844, -23.8654)
  spline S915 degree 3 poles (129.844, -23.8654) (129.844, -23.839) (129.8175, -23.8654) (129.844, -23.8654) knots 0 0 0 0 1 1 1 1
  line L1192 (129.844, -23.8654) -> (130.2144, -23.8654)
  spline S916 degree 3 poles (130.2144, -23.8654) (130.229, -23.8654) (130.2409, -23.8535) (130.2409, -23.839) knots 0 0 0 0 1 1 1 1
  line L1193 (130.2409, -23.839) -> (130.2409, -22.2515)
  spline S917 degree 3 poles (130.2409, -22.2515) (130.2409, -22.2369) (130.229, -22.225) (130.2144, -22.225) knots 0 0 0 0 1 1 1 1
  line L1194 (130.2144, -22.225) -> (129.844, -22.225)
  spline S918 degree 3 poles (129.844, -22.225) (129.8175, -22.225) (129.844, -22.2515) (129.844, -22.225) knots 0 0 0 0 1 1 1 1
  line L1195 (129.844, -22.225) -> (129.844, -20.6904)
  spline S919 degree 3 poles (129.844, -20.6904) (129.844, -20.664) (129.8175, -20.6904) (129.844, -20.6904) knots 0 0 0 0 1 1 1 1
  line L1196 (129.844, -20.6904) -> (130.2144, -20.6904)
  spline S920 degree 3 poles (130.2144, -20.6904) (130.229, -20.6904) (130.2409, -20.6785) (130.2409, -20.664) knots 0 0 0 0 1 1 1 1
  line L1197 (130.2409, -20.664) -> (130.2409, -19.0765)
  spline S921 degree 3 poles (130.2409, -19.0765) (130.2409, -19.0619) (130.229, -19.05) (130.2144, -19.05) knots 0 0 0 0 1 1 1 1
  line L1198 (130.2144, -19.05) -> (129.844, -19.05)
  spline S922 degree 3 poles (129.844, -19.05) (129.8175, -19.05) (129.844, -19.0765) (129.844, -19.05) knots 0 0 0 0 1 1 1 1
  line L1199 (129.844, -19.05) -> (129.844, -17.5154)
  spline S923 degree 3 poles (129.844, -17.5154) (129.844, -17.489) (129.8175, -17.5154) (129.844, -17.5154) knots 0 0 0 0 1 1 1 1
  line L1200 (129.844, -17.5154) -> (130.2144, -17.5154)
  spline S924 degree 3 poles (130.2144, -17.5154) (130.229, -17.5154) (130.2409, -17.5035) (130.2409, -17.489) knots 0 0 0 0 1 1 1 1
  line L1201 (130.2409, -17.489) -> (130.2409, -15.9015)
  spline S925 degree 3 poles (130.2409, -15.9015) (130.2409, -15.8869) (130.229, -15.875) (130.2144, -15.875) knots 0 0 0 0 1 1 1 1
  line L1202 (130.2144, -15.875) -> (129.844, -15.875)
  spline S926 degree 3 poles (129.844, -15.875) (129.8175, -15.875) (129.844, -15.9015) (129.844, -15.875) knots 0 0 0 0 1 1 1 1
  line L1203 (129.844, -15.875) -> (129.844, -14.3404)
  spline S927 degree 3 poles (129.844, -14.3404) (129.844, -14.314) (129.8175, -14.3404) (129.844, -14.3404) knots 0 0 0 0 1 1 1 1
  line L1204 (129.844, -14.3404) -> (130.2144, -14.3404)
  spline S928 degree 3 poles (130.2144, -14.3404) (130.229, -14.3404) (130.2409, -14.3285) (130.2409, -14.314) knots 0 0 0 0 1 1 1 1
  line L1205 (130.2409, -14.314) -> (130.2409, -12.7265)
  spline S929 degree 3 poles (130.2409, -12.7265) (130.2409, -12.7119) (130.229, -12.7) (130.2144, -12.7) knots 0 0 0 0 1 1 1 1
  line L1206 (130.2144, -12.7) -> (129.844, -12.7)
  spline S930 degree 3 poles (129.844, -12.7) (129.8175, -12.7) (129.844, -12.7265) (129.844, -12.7) knots 0 0 0 0 1 1 1 1
  line L1207 (129.844, -12.7) -> (129.844, -11.1654)
  spline S931 degree 3 poles (129.844, -11.1654) (129.844, -11.139) (129.8175, -11.1654) (129.844, -11.1654) knots 0 0 0 0 1 1 1 1
  line L1208 (129.844, -11.1654) -> (130.2144, -11.1654)
  spline S932 degree 3 poles (130.2144, -11.1654) (130.229, -11.1654) (130.2409, -11.1535) (130.2409, -11.139) knots 0 0 0 0 1 1 1 1
  line L1209 (130.2409, -11.139) -> (130.2409, -9.5515)
  spline S933 degree 3 poles (130.2409, -9.5515) (130.2409, -9.5369) (130.229, -9.525) (130.2144, -9.525) knots 0 0 0 0 1 1 1 1
  line L1210 (130.2144, -9.525) -> (129.844, -9.525)
  spline S934 degree 3 poles (129.844, -9.525) (129.8175, -9.525) (129.844, -9.5515) (129.844, -9.525) knots 0 0 0 0 1 1 1 1
  line L1211 (129.844, -9.525) -> (129.844, -7.9904)
  spline S935 degree 3 poles (129.844, -7.9904) (129.844, -7.964) (129.8175, -7.9904) (129.844, -7.9904) knots 0 0 0 0 1 1 1 1
  line L1212 (129.844, -7.9904) -> (130.2144, -7.9904)
  spline S936 degree 3 poles (130.2144, -7.9904) (130.229, -7.9904) (130.2409, -7.9785) (130.2409, -7.964) knots 0 0 0 0 1 1 1 1
  line L1213 (130.2409, -7.964) -> (130.2409, -6.3765)
  spline S937 degree 3 poles (130.2409, -6.3765) (130.2409, -6.3619) (130.229, -6.35) (130.2144, -6.35) knots 0 0 0 0 1 1 1 1
  line L1214 (130.2144, -6.35) -> (129.844, -6.35)
  spline S938 degree 3 poles (129.844, -6.35) (129.8175, -6.35) (129.844, -6.3765) (129.844, -6.35) knots 0 0 0 0 1 1 1 1
  line L1215 (129.844, -6.35) -> (129.844, -3.466)
  spline S939 degree 3 poles (129.844, -3.466) (129.844, -3.4515) (129.8321, -3.4396) (129.8175, -3.4396) knots 0 0 0 0 1 1 1 1
  line L1216 (129.8175, -3.4396) -> (130.0017, -3.4396)
  line L1217 (130.0017, -3.4396) -> (128.5962, -3.4396)
  spline S940 degree 3 poles (128.5962, -3.4396) (128.5698, -3.4396) (128.5962, -3.466) (128.5962, -3.4396) knots 0 0 0 0 1 1 1 1
  line L1218 (128.5962, -3.4396) -> (128.5962, -2.6723)
  spline S941 degree 3 poles (128.5962, -2.6723) (128.5962, -2.6577) (128.5846, -2.6458) (128.5698, -2.6458) knots 0 0 0 0 1 1 1 1
  line L1219 (128.5698, -2.6458) -> (126.9823, -2.6458)
  spline S942 degree 3 poles (126.9823, -2.6458) (126.9677, -2.6458) (126.9558, -2.6577) (126.9558, -2.6723) knots 0 0 0 0 1 1 1 1
  line L1220 (126.9558, -2.6723) -> (126.9558, -3.4396)
  spline S943 degree 3 poles (126.9558, -3.4396) (126.9558, -3.466) (126.9823, -3.4396) (126.9558, -3.4396) knots 0 0 0 0 1 1 1 1
  line L1221 (126.9558, -3.4396) -> (125.5506, -3.4396)
  line L1222 (125.5506, -3.4396) -> (125.4461, -3.4396)
  spline S944 degree 3 poles (125.4461, -3.4396) (125.4315, -3.4396) (125.4196, -3.4515) (125.4196, -3.466) knots 0 0 0 0 1 1 1 1
  line L1223 (125.4196, -3.466) -> (125.4196, -6.3765)
  spline S945 degree 3 poles (125.4196, -6.3765) (125.4196, -6.391) (125.4315, -6.4029) (125.4461, -6.4029) knots 0 0 0 0 1 1 1 1
  line L1224 (125.4461, -6.4029) -> (125.625, -6.4029)
  spline S946 degree 3 poles (125.625, -6.4029) (125.6514, -6.4029) (125.625, -6.3765) (125.625, -6.4029) knots 0 0 0 0 1 1 1 1
  line L1225 (125.625, -6.4029) -> (125.625, -7.9375)
  spline S947 degree 3 poles (125.625, -7.9375) (125.625, -7.964) (125.6514, -7.9375) (125.625, -7.9375) knots 0 0 0 0 1 1 1 1
  line L1226 (125.625, -7.9375) -> (125.4461, -7.9375)
  spline S948 degree 3 poles (125.4461, -7.9375) (125.4315, -7.9375) (125.4196, -7.9494) (125.4196, -7.964) knots 0 0 0 0 1 1 1 1
  line L1227 (125.4196, -7.964) -> (125.4196, -9.5515)
  spline S949 degree 3 poles (125.4196, -9.5515) (125.4196, -9.566) (125.4315, -9.5779) (125.4461, -9.5779) knots 0 0 0 0 1 1 1 1
  line L1228 (125.4461, -9.5779) -> (125.625, -9.5779)
  spline S950 degree 3 poles (125.625, -9.5779) (125.6514, -9.5779) (125.625, -9.5515) (125.625, -9.5779) knots 0 0 0 0 1 1 1 1
  line L1229 (125.625, -9.5779) -> (125.625, -11.1125)
  spline S951 degree 3 poles (125.625, -11.1125) (125.625, -11.139) (125.6514, -11.1125) (125.625, -11.1125) knots 0 0 0 0 1 1 1 1
  line L1230 (125.625, -11.1125) -> (125.4461, -11.1125)
  spline S952 degree 3 poles (125.4461, -11.1125) (125.4315, -11.1125) (125.4196, -11.1244) (125.4196, -11.139) knots 0 0 0 0 1 1 1 1
  line L1231 (125.4196, -11.139) -> (125.4196, -12.7265)
  spline S953 degree 3 poles (125.4196, -12.7265) (125.4196, -12.741) (125.4315, -12.7529) (125.4461, -12.7529) knots 0 0 0 0 1 1 1 1
  line L1232 (125.4461, -12.7529) -> (125.625, -12.7529)
  spline S954 degree 3 poles (125.625, -12.7529) (125.6514, -12.7529) (125.625, -12.7265) (125.625, -12.7529) knots 0 0 0 0 1 1 1 1
  line L1233 (125.625, -12.7529) -> (125.625, -14.2875)
  spline S955 degree 3 poles (125.625, -14.2875) (125.625, -14.314) (125.6514, -14.2875) (125.625, -14.2875) knots 0 0 0 0 1 1 1 1
  line L1234 (125.625, -14.2875) -> (125.4461, -14.2875)
  spline S956 degree 3 poles (125.4461, -14.2875) (125.4315, -14.2875) (125.4196, -14.2994) (125.4196, -14.314) knots 0 0 0 0 1 1 1 1
  line L1235 (125.4196, -14.314) -> (125.4196, -15.9015)
  spline S957 degree 3 poles (125.4196, -15.9015) (125.4196, -15.916) (125.4315, -15.9279) (125.4461, -15.9279) knots 0 0 0 0 1 1 1 1
  line L1236 (125.4461, -15.9279) -> (125.625, -15.9279)
  spline S958 degree 3 poles (125.625, -15.9279) (125.6514, -15.9279) (125.625, -15.9015) (125.625, -15.9279) knots 0 0 0 0 1 1 1 1
  line L1237 (125.625, -15.9279) -> (125.625, -17.4625)
  spline S959 degree 3 poles (125.625, -17.4625) (125.625, -17.489) (125.6514, -17.4625) (125.625, -17.4625) knots 0 0 0 0 1 1 1 1
  line L1238 (125.625, -17.4625) -> (125.4461, -17.4625)
  spline S960 degree 3 poles (125.4461, -17.4625) (125.4315, -17.4625) (125.4196, -17.4744) (125.4196, -17.489) knots 0 0 0 0 1 1 1 1
  line L1239 (125.4196, -17.489) -> (125.4196, -19.0765)
  spline S961 degree 3 poles (125.4196, -19.0765) (125.4196, -19.091) (125.4315, -19.1029) (125.4461, -19.1029) knots 0 0 0 0 1 1 1 1
  line L1240 (125.4461, -19.1029) -> (125.625, -19.1029)
  spline S962 degree 3 poles (125.625, -19.1029) (125.6514, -19.1029) (125.625, -19.0765) (125.625, -19.1029) knots 0 0 0 0 1 1 1 1
  line L1241 (125.625, -19.1029) -> (125.625, -20.6375)
  spline S963 degree 3 poles (125.625, -20.6375) (125.625, -20.664) (125.6514, -20.6375) (125.625, -20.6375) knots 0 0 0 0 1 1 1 1
  line L1242 (125.625, -20.6375) -> (125.4461, -20.6375)
  spline S964 degree 3 poles (125.4461, -20.6375) (125.4315, -20.6375) (125.4196, -20.6494) (125.4196, -20.664) knots 0 0 0 0 1 1 1 1
  line L1243 (125.4196, -20.664) -> (125.4196, -22.2515)
  spline S965 degree 3 poles (125.4196, -22.2515) (125.4196, -22.266) (125.4315, -22.2779) (125.4461, -22.2779) knots 0 0 0 0 1 1 1 1
  line L1244 (125.4461, -22.2779) -> (125.625, -22.2779)
  spline S966 degree 3 poles (125.625, -22.2779) (125.6514, -22.2779) (125.625, -22.2515) (125.625, -22.2779) knots 0 0 0 0 1 1 1 1
  line L1245 (125.625, -22.2779) -> (125.625, -23.8125)
  spline S967 degree 3 poles (125.625, -23.8125) (125.625, -23.839) (125.6514, -23.8125) (125.625, -23.8125) knots 0 0 0 0 1 1 1 1
  line L1246 (125.625, -23.8125) -> (125.4461, -23.8125)
  spline S968 degree 3 poles (125.4461, -23.8125) (125.4315, -23.8125) (125.4196, -23.8244) (125.4196, -23.839) knots 0 0 0 0 1 1 1 1
  line L1247 (125.4196, -23.839) -> (125.4196, -25.4265)
  spline S969 degree 3 poles (125.4196, -25.4265) (125.4196, -25.441) (125.4315, -25.4529) (125.4461, -25.4529) knots 0 0 0 0 1 1 1 1
  line L1248 (125.4461, -25.4529) -> (125.625, -25.4529)
  spline S970 degree 3 poles (125.625, -25.4529) (125.6514, -25.4529) (125.625, -25.4265) (125.625, -25.4529) knots 0 0 0 0 1 1 1 1
  line L1249 (125.625, -25.4529) -> (125.625, -26.9875)
  spline S971 degree 3 poles (125.625, -26.9875) (125.625, -27.014) (125.6514, -26.9875) (125.625, -26.9875) knots 0 0 0 0 1 1 1 1
  line L1250 (125.625, -26.9875) -> (125.4461, -26.9875)
  spline S972 degree 3 poles (125.4461, -26.9875) (125.4315, -26.9875) (125.4196, -26.9994) (125.4196, -27.014) knots 0 0 0 0 1 1 1 1
  line L1251 (125.4196, -27.014) -> (125.4196, -29.9244)
  spline S973 degree 3 poles (125.4196, -29.9244) (125.4196, -29.9389) (125.4315, -29.9508) (125.4461, -29.9508) knots 0 0 0 0 1 1 1 1
  line L1252 (125.4461, -29.9508) -> (125.5506, -29.9508)
  line L1253 (130.8769, -29.9508) -> (132.2821, -29.9508)
  spline S974 degree 3 poles (132.2821, -29.9508) (132.3086, -29.9508) (132.2821, -29.9244) (132.2821, -29.9508) knots 0 0 0 0 1 1 1 1
  line L1254 (132.2821, -29.9508) -> (132.2821, -30.7181)
  spline S975 degree 3 poles (132.2821, -30.7181) (132.2821, -30.7327) (132.294, -30.7446) (132.3086, -30.7446) knots 0 0 0 0 1 1 1 1
  line L1255 (132.3086, -30.7446) -> (133.8961, -30.7446)
  spline S976 degree 3 poles (133.8961, -30.7446) (133.9109, -30.7446) (133.9226, -30.7327) (133.9226, -30.7181) knots 0 0 0 0 1 1 1 1
  line L1256 (133.9226, -30.7181) -> (133.9226, -29.9508)
  spline S977 degree 3 poles (133.9226, -29.9508) (133.9226, -29.9244) (133.8961, -29.9508) (133.9226, -29.9508) knots 0 0 0 0 1 1 1 1
  line L1257 (133.9226, -29.9508) -> (135.328, -29.9508)
  line L1258 (135.328, -29.9508) -> (135.1439, -29.9508)
  spline S978 degree 3 poles (135.1439, -29.9508) (135.1584, -29.9508) (135.1703, -29.9389) (135.1703, -29.9244) knots 0 0 0 0 1 1 1 1
  line L1259 (135.1703, -29.9244) -> (135.1703, -27.0404)
  spline S979 degree 3 poles (135.1703, -27.0404) (135.1703, -27.014) (135.1439, -27.0404) (135.1703, -27.0404) knots 0 0 0 0 1 1 1 1
  line L1260 (135.1703, -27.0404) -> (135.5408, -27.0404)
  spline S980 degree 3 poles (135.5408, -27.0404) (135.5553, -27.0404) (135.5672, -27.0285) (135.5672, -27.014) knots 0 0 0 0 1 1 1 1
  line L1261 (135.5672, -27.014) -> (135.5672, -25.4265)
  spline S981 degree 3 poles (135.5672, -25.4265) (135.5672, -25.4119) (135.5553, -25.4) (135.5408, -25.4) knots 0 0 0 0 1 1 1 1
  line L1262 (135.5408, -25.4) -> (135.1703, -25.4)
  spline S982 degree 3 poles (135.1703, -25.4) (135.1439, -25.4) (135.1703, -25.4265) (135.1703, -25.4) knots 0 0 0 0 1 1 1 1
  line L1263 (135.1703, -25.4) -> (135.1703, -23.8654)
  spline S983 degree 3 poles (135.1703, -23.8654) (135.1703, -23.839) (135.1439, -23.8654) (135.1703, -23.8654) knots 0 0 0 0 1 1 1 1
  line L1264 (135.1703, -23.8654) -> (135.5408, -23.8654)
  spline S984 degree 3 poles (135.5408, -23.8654) (135.5553, -23.8654) (135.5672, -23.8535) (135.5672, -23.839) knots 0 0 0 0 1 1 1 1
  line L1265 (135.5672, -23.839) -> (135.5672, -22.2515)
  spline S985 degree 3 poles (135.5672, -22.2515) (135.5672, -22.2369) (135.5553, -22.225) (135.5408, -22.225) knots 0 0 0 0 1 1 1 1
  line L1266 (135.5408, -22.225) -> (135.1703, -22.225)
  spline S986 degree 3 poles (135.1703, -22.225) (135.1439, -22.225) (135.1703, -22.2515) (135.1703, -22.225) knots 0 0 0 0 1 1 1 1
  line L1267 (135.1703, -22.225) -> (135.1703, -20.6904)
  spline S987 degree 3 poles (135.1703, -20.6904) (135.1703, -20.664) (135.1439, -20.6904) (135.1703, -20.6904) knots 0 0 0 0 1 1 1 1
  line L1268 (135.1703, -20.6904) -> (135.5408, -20.6904)
  spline S988 degree 3 poles (135.5408, -20.6904) (135.5553, -20.6904) (135.5672, -20.6785) (135.5672, -20.664) knots 0 0 0 0 1 1 1 1
  line L1269 (135.5672, -20.664) -> (135.5672, -19.0765)
  spline S989 degree 3 poles (135.5672, -19.0765) (135.5672, -19.0619) (135.5553, -19.05) (135.5408, -19.05) knots 0 0 0 0 1 1 1 1
  line L1270 (135.5408, -19.05) -> (135.1703, -19.05)
  spline S990 degree 3 poles (135.1703, -19.05) (135.1439, -19.05) (135.1703, -19.0765) (135.1703, -19.05) knots 0 0 0 0 1 1 1 1
  line L1271 (135.1703, -19.05) -> (135.1703, -17.5154)
  spline S991 degree 3 poles (135.1703, -17.5154) (135.1703, -17.489) (135.1439, -17.5154) (135.1703, -17.5154) knots 0 0 0 0 1 1 1 1
  line L1272 (135.1703, -17.5154) -> (135.5408, -17.5154)
  spline S992 degree 3 poles (135.5408, -17.5154) (135.5553, -17.5154) (135.5672, -17.5035) (135.5672, -17.489) knots 0 0 0 0 1 1 1 1